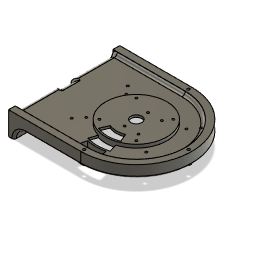
base v15 (Autodesk Fusion 360 design; units mm, degrees)
Autodesk Fusion 360 part; units mm, degrees
note: some values were not read from the file. Chosen so that the rebuilt part matches the saved one: which face or edge a step refers to; which pieces of a blend or face edit are solid. Set by a fixed rule: which sketch regions a step uses.
sketch "スケッチ1" plane through (0, 0, 0) normal (0, 1, 0) x (1, 0, 0)
  circle A0 centre (0, 0) radius 44
  line L0 (0, -123.2067) -> (0, 133.3084) construction
  line L1 (-140.7912, 0) -> (211.312, 0) construction
  circle A1 centre (0, 0) radius 35
  circle A2 centre (0, 0) radius 26
  circle A3 centre (0, 0) radius 5
  line L2 (12.5, -10.5) -> (0, -10.5) construction
  line L3 (0, -10.5) -> (0, 10.5) construction
  line L4 (0, 10.5) -> (12.5, 10.5) construction
  line L5 (12.5, 10.5) -> (12.5, -10.5) construction
  circle A4 centre (0, 10.5) radius 1
  circle A5 centre (12.5, 10.5) radius 1
  circle A6 centre (12.5, -10.5) radius 1
  circle A7 centre (0, -10.5) radius 1
  circle A8 centre (0, 0) radius 45.5
  circle A9 centre (0, 0) radius 36.5
  circle A10 centre (0, 0) radius 27.5
  circle A11 centre (0, 0) radius 50
  line L6 (0, -50) -> (-60, -50)
  line L7 (0, 50) -> (-60, 50)
  line L8 (-60, -50) -> (-60, 50)
  circle A12 centre (0, 0) radius 18 construction
  arc A13 (-6.9231, -16.6154) -> (6.9231, -16.6154) centre (0, 0) ccw
  line L9 (6.9231, -16.6154) -> (10, -24)
  line L10 (-6.9231, -16.6154) -> (-10, -24)
  line L11 (-7.8571, -26.3537) -> (-10, -33.541)
  line L12 (-8.2955, -35.5448) -> (-10, -42.8486)
  line L13 (10, -42.8486) -> (8.2955, -35.5448)
  line L14 (10, -33.541) -> (7.8571, -26.3537)
  line L15 (-60, -50) -> (-65, -50)
  line L16 (-65, -50) -> (-65, 50)
  line L17 (-65, 50) -> (-60, 50)
  line L18 (-60, 50) -> (-60, -50)
  line L19 (-65, -44) -> (-23.7487, -44)
  line L20 (-65, 44) -> (-23.7487, 44)
  circle A14 centre (0, 0) radius 47 construction
  circle A15 centre (0, -47) radius 3
  circle A16 centre (47, 0) radius 3
  circle A17 centre (0, 47) radius 3
  circle A18 centre (0, -47) radius 2.25
  circle A19 centre (0, -47) radius 1.15
  circle A20 centre (47, 0) radius 2.25
  circle A21 centre (47, 0) radius 1.15
  circle A22 centre (0, 47) radius 2.25
  circle A23 centre (0, 47) radius 1.15
  line L21 (-60, -6.25) -> (-65, -6.25) construction
  line L22 (-65, -5.25) -> (-60, -5.25) construction
  line L23 (-60, 5.25) -> (-65, 5.25) construction
  line L24 (-65, 6.25) -> (-60, 6.25) construction
  line L25 (-62.5, 5.25) -> (-62.5, -5.25)
  line L26 (-62.5, -5.25) -> (-65, -6.25)
  line L27 (-62.5, 5.25) -> (-65, 6.25)
  circle A24 centre (0, 0) radius 41.5 construction
  circle A25 centre (0, 0) radius 32.5 construction
  circle A26 centre (0, 0) radius 23.5 construction
  line L28 (10, -48.9898) -> (10, 48.9898) construction
  line L29 (-10, -48.9898) -> (-10, 48.9898) construction
  line L30 (10, -33.541) -> (0, 0) construction
  line L31 (-10, -33.541) -> (0, 0) construction
  line L32 (10, -24) -> (0, 0) construction
  line L33 (-10, -24) -> (0, 0) construction
  line L34 (10, -42.8486) -> (0, 0) construction
  line L35 (-10, -42.8486) -> (0, 0) construction
  line L36 (32.9242, -25.2636) -> (-32.9242, 25.2636) construction
  line L37 (-32.9242, -25.2636) -> (32.9242, 25.2636) construction
  line L38 (27.0228, -18.056) -> (-27.0228, 18.056) construction
  line L39 (27.0228, 18.056) -> (-27.0228, -18.056) construction
  line L40 (16.617, -16.617) -> (-16.617, 16.617) construction
  line L41 (16.617, 16.617) -> (-16.617, -16.617) construction
  circle A27 centre (32.9242, -25.2636) radius 1
  circle A28 centre (27.0228, -18.056) radius 1
  circle A29 centre (16.617, -16.617) radius 1
  circle A30 centre (-27.0228, -18.056) radius 1
  circle A31 centre (-32.9242, -25.2636) radius 1
  circle A32 centre (-16.617, -16.617) radius 1
  circle A33 centre (32.9242, 25.2636) radius 1
  circle A34 centre (27.0228, 18.056) radius 1
  circle A35 centre (16.617, 16.617) radius 1
  circle A36 centre (-16.617, 16.617) radius 1
  circle A37 centre (-27.0228, 18.056) radius 1
  circle A38 centre (-32.9242, 25.2636) radius 1
  line L42 (-23.7487, -44) -> (0, -44)
  line L43 (-23.7487, 44) -> (0, 44)
  dimension "d1" = 88
  dimension "d2" = 70
  dimension "d3" = 52
  dimension "d4" = 10
  dimension "d5" = 10.5
  dimension "d6" = 21
  dimension "d8" = 12.5
  dimension "d9" = 2
  dimension "d10" = 2
  dimension "d11" = 2
  dimension "d12" = 2
  dimension "d13" = 1.5
  dimension "d14" = 1.5
  dimension "d15" = 1.5
  dimension "d22" = 100
  dimension "d23" = 60
  dimension "d28" = 36
  dimension "d29" = 5
  dimension "d30" = 6
  dimension "d31" = 6
  dimension "d32" = 94
  dimension "d33" = 6
  dimension "d34" = 6
  dimension "d35" = 6
  dimension "d36" = 4.5
  dimension "d37" = 2.3
  dimension "d38" = 4.5
  dimension "d39" = 2.3
  dimension "d40" = 4.5
  dimension "d41" = 2.3
  dimension "d78" = 5.25
  dimension "d79" = 1
  dimension "d80" = 10.5
  dimension "d81" = 12.5
  dimension "d82" = 2.5
  dimension "d90" = 10
  dimension "d91" = 20
  dimension "d92" = 52.5
  dimension "d93" = 56.25
  dimension "d94" = 45
  dimension "d95" = 52.5
  dimension "d96" = 56.25
  dimension "d97" = 45
  dimension "d98" = 2
  dimension "d99" = 2
  dimension "d100" = 2
  dimension "d101" = 2
  dimension "d102" = 2
  dimension "d103" = 2
  dimension "d104" = 47
  dimension "d105" = 65
  dimension "d106" = 83
  dimension "d107" = 2
  dimension "d108" = 2
  dimension "d109" = 2
  dimension "d110" = 2
  dimension "d111" = 2
  dimension "d112" = 2
  constraint coincident A0.centre A1.centre
  constraint vertical L0
  constraint perpendicular L0 L1
  constraint concentric A0 A1
  constraint concentric A0 A2
  constraint concentric A1 A3
  constraint horizontal L2
  constraint vertical L3
  constraint horizontal L4
  constraint vertical L5
  constraint coincident L3.end L4.start
  constraint coincident L4.end L5.start
  constraint coincident L2.start L5.end
  constraint coincident L2.end L3.start
  constraint concentric A1 A11
  constraint coincident A11 L6.start
  constraint coincident L0 L6.start
  constraint perpendicular L0 L6
  constraint coincident A11 L7.start
  constraint coincident L0 L7.start
  constraint perpendicular L0 L7
  constraint concentric A0 A12
  constraint coincident A12 A13.end
  constraint coincident A2 L9.end
  constraint coincident A2 L10.end
  constraint coincident A10 L11.start
  constraint coincident A1 L11.end
  constraint coincident A9 L12.start
  constraint coincident A0 L12.end
  constraint coincident A0 L13.start
  constraint coincident A9 L13.end
  constraint coincident A1 L14.start
  constraint coincident A10 L14.end
  constraint parallel L0 L8
  constraint horizontal L15
  constraint vertical L16
  constraint horizontal L17
  constraint vertical L18
  constraint coincident L16 L19.start
  constraint coincident A11 L19.end
  constraint perpendicular L16 L19
  constraint coincident L16 L20.start
  constraint coincident A11 L20.end
  constraint perpendicular L16 L20
  constraint concentric A12 A14
  constraint coincident L0 A15.centre
  constraint coincident A14 A15.centre
  constraint coincident L1 A16.centre
  constraint coincident A14 A16.centre
  constraint coincident L0 A17.centre
  constraint coincident A14 A17.centre
  constraint concentric A15 A18
  constraint concentric A15 A19
  constraint concentric A16 A20
  constraint concentric A16 A21
  constraint concentric A17 A22
  constraint concentric A22 A23
  constraint coincident L8 L21.start
  constraint coincident L16 L21.end
  constraint perpendicular L16 L21
  constraint coincident L16 L22.start
  constraint coincident L18 L22.end
  constraint perpendicular L18 L22
  constraint coincident L8 L23.start
  constraint coincident L16 L23.end
  constraint perpendicular L16 L23
  constraint coincident L16 L24.start
  constraint coincident L18 L24.end
  constraint perpendicular L18 L24
  constraint midpoint L23 L25.start
  constraint perpendicular L1 L25
  constraint midpoint L22 L25.end
  constraint concentric A2 A24
  constraint concentric A0 A25
  constraint concentric A1 A26
  constraint vertical L28
  constraint perpendicular L7 L29
  constraint coincident A11 L28.start
  constraint coincident A11 L29.start
  constraint coincident A11 L29.end
  constraint coincident A11 L28.end
  constraint coincident L13.start L28
  constraint coincident L12.end L29
  constraint coincident L14.start L28
  constraint coincident L11.end L29
  constraint coincident L9.end L28
  constraint coincident L10.end L29
  constraint collinear L12 L35
  constraint collinear L11 L31
  constraint collinear L10 L33
  constraint collinear L9 L32
  constraint collinear L14 L30
  constraint collinear L13 L34
  constraint coincident A24 L36.start
  constraint coincident A24 L36.end
  constraint coincident A24 L37.start
  constraint coincident A24 L37.end
  constraint coincident A25 L38.start
  constraint coincident A25 L38.end
  constraint coincident A25 L39.start
  constraint coincident A25 L39.end
  constraint coincident A26 L40.start
  constraint coincident A26 L40.end
  constraint coincident A26 L41.end
  constraint coincident A0.centre L36
  constraint coincident A0.centre L38
  constraint coincident A0.centre L40
  constraint coincident A0.centre L41
  constraint coincident A0.centre L37
  constraint coincident A0.centre L39
  constraint coincident L36.start A27.centre
  constraint coincident L38.start A28.centre
  constraint coincident L40.start A29.centre
  constraint coincident L39.end A30.centre
  constraint coincident L37.start A31.centre
  constraint coincident L41.end A32.centre
  constraint coincident L37.end A33.centre
  constraint coincident L39.start A34.centre
  constraint coincident A26 L41.start
  constraint coincident L41.start A35.centre
  constraint coincident L40.end A36.centre
  constraint coincident L38.end A37.centre
  constraint coincident L36.end A38.centre
  constraint coincident A15 L42.end
  constraint parallel L19 L42
  constraint coincident A17 L43.end
  constraint parallel L20 L43
  constraint collinear L0 L3
  measures "d1" diameter of A0
  measures "d2" diameter of A1
  measures "d3" diameter of A2
  measures "d4" diameter of A3
  measures "d5" distance of L1 L2
  measures "d6" distance of L2 L4
  measures "d8" distance of L3 L5
  measures "d9" diameter of A4
  measures "d10" diameter of A5
  measures "d11" diameter of A6
  measures "d12" diameter of A7
  measures "d22" diameter of A11
  measures "d23" distance of L6.start L6.end
  measures "d28" diameter of A12
  measures "d29" distance of L6.end L15.end
  measures "d30" distance of L6 L19
  measures "d31" distance of L7 L20
  measures "d32" diameter of A14
  measures "d33" diameter of A15
  measures "d34" diameter of A16
  measures "d35" diameter of A17
  measures "d36" diameter of A18
  measures "d37" diameter of A19
  measures "d38" diameter of A20
  measures "d39" diameter of A21
  measures "d40" diameter of A22
  measures "d41" diameter of A23
  measures "d78" distance of L1 L22
  measures "d79" distance of L21 L22
  measures "d80" distance of L22 L23
  measures "d81" distance of L21 L24
  measures "d82" distance of L16 L25
  measures "d90" distance of L0 L28
  measures "d91" distance of L28 L29
  measures "d92" angle of L0 L36
  measures "d93" angle of L0 L38
  measures "d94" angle of L0 L40
  measures "d95" angle of L0 L37
  measures "d96" angle of L0 L39
  measures "d97" angle of L0 L41
  measures "d98" diameter of A27
  measures "d99" diameter of A28
  measures "d100" diameter of A29
  measures "d101" diameter of A30
  measures "d102" diameter of A31
  measures "d103" diameter of A32
  measures "d104" diameter of A26
  measures "d105" diameter of A25
  measures "d106" diameter of A24
  measures "d107" diameter of A33
  measures "d108" diameter of A34
  measures "d109" diameter of A35
  measures "d110" diameter of A36
  measures "d111" diameter of A37
  measures "d112" diameter of A38
extrude "押し出し1" add sketch "スケッチ1" along normal blind 2 contours A8 A11 A16 A17 | A8 A11 A15 A16 | A8 A11 A17 L43 | A8 A11 L42 L43 | A8 A11 A15 L42 | A11 L8 L18 L19 L20 makes body 1 at (-55.1272, 0, 1.0929)
extrude "押し出し2" add sketch "スケッチ1" along normal blind 5 contours A0 A8 A15 A16 | A0 A8 A16 A17 | A8 A16 A20 | A8 A17 L43 | A8 A17 A22 | A0 A8 L42 L43 | A8 A16 A20 | A8 A11 A16 A17 | A8 A11 A15 A16 | A8 A17 A22 | A8 A11 A17 L43 | A8 A11 L42 L43 | A8 A15 A18 | A8 A15 L42 | A8 A15 A18 | A11 L7 L8 L18 L20 | A8 A11 A15 L42 | A11 L6 L8 L18 L19 | L8 L16 L17 L18 L20 | L8 L16 L18 L19 L20 L25 L26 L27 | L8 L15 L16 L18 L19 | L16 L25 L26 L27 bodies 1
extrude "押し出し3" add sketch "スケッチ1" along normal blind 2 from surface at 3 contours A0 A9 L12 L13 | A0 A8 L42 L43 | A8 A11 L42 L43 | A11 L8 L18 L19 L20 picked at (35.2878, -19.7128) bodies 1
extrude "押し出し4" add sketch "スケッチ1" along normal blind 5 from surface at 3 contours A0 A9 L12 L13 | A0 A8 L42 L43 | A8 A11 L42 L43 | A9 | A11 L8 L18 L19 L20 picked at (35.2878, -19.7128) bodies 1
extrude "押し出し5" add sketch "スケッチ1" along normal blind 2 from surface at 6 contours A1 A10 L11 L14 picked at (-23.496, 20.8927) bodies 1
extrude "押し出し6" add sketch "スケッチ1" along normal blind 5 from surface at 6 contours A10 bodies 1
extrude "押し出し7" add sketch "スケッチ1" along normal blind 2 from surface at 9 contours A8 A20 | A8 A20 | A8 A22 | A8 A22 | A8 A18 | A8 A18 | A2 A13 L9 L10 picked at (17.2436, 0) bodies 1 makes body 2 at (2.2388, 10.3333, -47.224) makes body 3 at (47.7166, 9.6667, -2.1328) makes body 4 at (2.2388, 10.3333, 46.776)
extrude "押し出し8" add sketch "スケッチ1" against normal blind 10 contours L8 L16 L17 L18 L20 | L8 L16 L18 L19 L20 L25 L26 L27 | L8 L15 L16 L18 L19 | L16 L25 L26 L27 bodies 1
fillet "フィレット1" radius 10 1 edges at (-60, 0, 0) on bodies 1
sketch "スケッチ2" plane through (-65, 0, 0) normal (-1, 0, 0) x (0, 0, 1)
  line L0 (50, -10) -> (50, 5)
  line L1 (50, 5) -> (-50, 5)
  line L2 (-50, 5) -> (-50, -10)
  line L3 (-50, -10) -> (50, -10)
  line L4 (-50, 5) -> (50, 5)
  line L5 (50, 5) -> (50, -10)
  line L6 (50, -10) -> (-50, -10)
  line L7 (-50, -10) -> (-50, 5)
  line L8 (-59.5301, -2.5) -> (54.6644, -2.5) construction
  line L9 (-30, 17.3298) -> (-30, -19.2966) construction
  line L10 (30, 17.3298) -> (30, -23.1694) construction
  circle A0 centre (-30, -2.5) radius 1.3
  circle A1 centre (30, -2.9198) radius 1.3
  line L11 (-5, 5) -> (-5, -10)
  line L12 (5, 5) -> (5, -10)
  line L13 (0, 28.6511) -> (0, -23.9207) construction
  dimension "d67" = 15
  dimension "d68" = 100
  dimension "d69" = 20
  dimension "d70" = 20
  dimension "d71" = 7.5
  dimension "d72" = 2.6
  dimension "d73" = 2.6
  dimension "d76" = 5
  dimension "d77" = 10
  constraint horizontal L4
  constraint vertical L5
  constraint horizontal L6
  constraint vertical L7
  constraint coincident L0.start L3.end
  constraint coincident L1.end L2.start
  constraint perpendicular L5 L8
  constraint perpendicular L6 L9
  constraint perpendicular L6 L10
  constraint coincident L8 A0.centre
  constraint coincident L9 A0.centre
  constraint midpoint L10 A1.centre
  constraint coincident L4 L11.start
  constraint coincident L6 L11.end
  constraint perpendicular L6 L11
  constraint coincident L4 L12.start
  constraint coincident L6 L12.end
  constraint perpendicular L6 L12
  constraint perpendicular L4 L13
  measures "d67" distance of L4 L6
  measures "d68" distance of L5 L7
  measures "d69" distance of L7 L9
  measures "d70" distance of L5 L10
  measures "d71" distance of L6 L8
  measures "d72" diameter of A0
  measures "d73" diameter of A1
  measures "d76" distance of L12 L13
  measures "d77" distance of L11 L12
extrude "押し出し9" cut sketch "スケッチ2" against normal blind 5 contours A0 | A1 bodies 1
extrude "押し出し10" cut sketch "スケッチ1" along normal up to surface (5 mm away) and the other way up to surface (10 mm away) contours L16 L25 L26 L27 bodies 1
extrude "押し出し11" add sketch "スケッチ1" along normal up to surface (11 mm away) contours A0 A8 A15 A16 | A0 A8 A16 A17 | A8 A16 A20 | A8 A17 L43 | A8 A17 A22 | A8 A16 A20 | A8 A11 A16 A17 | A8 A11 A15 A16 | A8 A17 A22 | A8 A11 A17 L43 | A8 A15 A18 | A8 A15 L42 | A8 A15 A18 | A11 L7 L8 L18 L20 | A8 A11 A15 L42 | A11 L6 L8 L18 L19 | L8 L16 L17 L18 L20 | L8 L15 L16 L18 L19 bodies 1 2 3 4
fillet "フィレット3" radius 2 5 edges at (-57.0711, -2.9289, 50) (-25, 0, 50) (50, 0, 0) (-25, 0, -50) (-57.0711, -2.9289, -50) on bodies 1
extrude "押し出し12" add sketch "スケッチ1" along normal up to surface (8 mm away) contours L8 L16 L18 L19 L20 L25 L26 L27 bodies 1
fillet "フィレット4" radius 4 5 edges at (-65, 8, 25.125) (-62.5, 8, 0) (-65, 8, -25.125) (-63.75, 8, -5.75) (-63.75, 8, 5.75) on bodies 1
fillet "フィレット5" radius 2.9 3 edges at (43.7112, 8, -5.033) (-30.5, 8, -44) (-63.8284, 6.8284, -44) on bodies 1
fillet "フィレット6" radius 2.95 2 edges at (-30.5, 8, 44) (-63.8284, 6.8284, 44) on bodies 1
equation "d90 = d91 / 2"
equation "d95 = d92"
equation "d96 = d93"
equation "d97 = d94"
